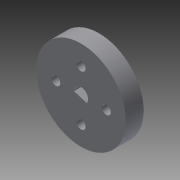
# Autodesk Inventor part: stepperShaftCollar_RB01
Saved by Autodesk Inventor 2013 (Build 170138000, 138)
## iProperties
Created: 2014-06-14
Part Number: stepperShaftCollar_RB01
Material: Generic
Document SubType Name: Modeling
Designer: Byron
Density: 1 g/cm^3
Author: Byron
Autodesk Inventor part; units mm, degrees
ref_plane "YZ Plane" through (0, 0, 0) normal (1, 0, 0) x (0, 1, 0)
ref_plane "XZ Plane" through (0, 0, 0) normal (0, 1, 0) x (-1, 0, 0)
ref_plane "XY Plane" through (0, 0, 0) normal (0, 0, 1) x (1, 0, 0)
sketch "Sketch1" plane through (0, 0, 0) normal (0, 0, 1) x (1, 0, 0)
  circle A0 centre (-17.1376, -0.8341) radius 15.875
  circle A1 centre (-17.1376, -9.7932) radius 1.5875
  circle A2 centre (-8.1786, -0.8341) radius 1.5875
  circle A3 centre (-17.1376, 8.1249) radius 1.5875
  circle A4 centre (-26.0966, -0.8341) radius 1.5875
  line L0 (-19.6376, -0.8341) -> (-15.1013, -2.2845)
  arc A5 (-15.1013, -2.2845) -> (-19.6376, -0.8341) centre (-17.1376, -0.8341) ccw
  arc A6 (-15.1013, -2.2845) -> (-19.6376, -0.8341) centre (-17.1376, -0.8341) ccw
  arc A7 (-15.1013, -2.2845) -> (-19.6376, -0.8341) centre (-17.1376, -0.8341) ccw
  point P0 (0, 0)
  dimension "d0" = 5
  dimension "d1" = 31.75
  dimension "d2" = 3.175
  dimension "d5" = 360
  constraints: 8 centre point, 6 point on circle, 2 end point, 9 other
  measures "d0" diameter of A5
  measures "d1" diameter of A0
  measures "d2" diameter of A1
extrude "Extrusion1" add sketch "Sketch1" along normal blind 6.35 contours A0 | A5 L0
sketch "Sketch2" plane through (-17.1376, -0.8341, 0) normal (0, 0, -1) x (-1, 0, 0)
  line L0 (2.5, 0) -> (-2.0363, -1.4504)
  arc A0 (2.5, 0) -> (-2.0363, -1.4504) centre (0, 0) ccw
  point P0 (-17.1376, 0.8341)
  constraints: 2 end point, 2 point on circle, 1 centre point
extrude "Extrusion2" cut sketch "Sketch2" against normal through all
body "Solid1"
